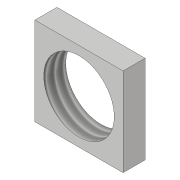
# Autodesk Inventor part: DC MOTOR NUT FOR CAPPING SYSTEM
Saved by Autodesk Inventor 2019 (Build 230136000, 136)
## iProperties
Created: 2019-10-13
Part Number: DC MOTOR NUT FOR CAPPING SYSTEM
Material: Generic
Document SubType Name: Modeling
Designer: Admin
Density: 1 g/cm^3
Appearance: Default
Author: Admin
Autodesk Inventor part; units mm, degrees
ref_plane "YZ Plane" through (0, 0, 0) normal (1, 0, 0) x (0, 1, 0)
ref_plane "XZ Plane" through (0, 0, 0) normal (0, 1, 0) x (-1, 0, 0)
ref_plane "XY Plane" through (0, 0, 0) normal (0, 0, 1) x (1, 0, 0)
sketch "Sketch1" plane through (0, 0, 0) normal (0, 0, 1) x (1, 0, 0)
  line L0 (0, 0) -> (20, 0)
  line L1 (20, 0) -> (20, 20)
  line L2 (20, 20) -> (0, 20)
  line L3 (0, 20) -> (0, 0)
  dimension "d0" = 20
  dimension "d1" = 20
  constraints: 8 end point, 2 parallel, 1 horizontal, 1 perpendicular
  measures "d0" distance of L2.end L1.end
  measures "d1" distance of L1.end L0.end
extrude "Extrusion1" add sketch "Sketch1" along normal blind 5
sketch "Sketch2" plane through (0, 0, 5) normal (0, 0, 1) x (1, 0, 0)
  line L0 (0, 0) -> (10, 0)
  line L1 (0, 0) -> (20, 0) projected
  line L2 (10, 0) -> (10, 10)
  circle A0 centre (10, 10) radius 8
  dimension "d4" = 10
  dimension "d5" = 10
  dimension "d6" = 16
  constraints: 4 end point, 1 centre point, 1 coincident, 1 midpoint, 1 perpendicular
  measures "d4" distance of L0.start L0.end
  measures "d5" distance of L0.end L2.end
  measures "d6" diameter of A0
extrude "Extrusion2" cut sketch "Sketch2" against normal through all
thread "Thread1" size "M16x2" class "6H" standard "ANSI Metric M Profile" full length
body "Solid1"
